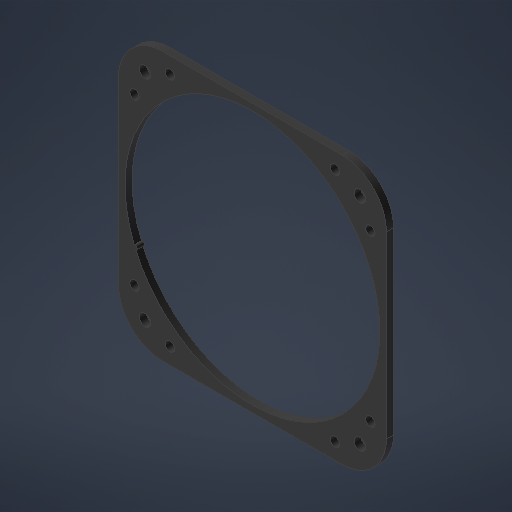
# Autodesk Inventor part: stator_center_00_alu
Saved by Autodesk Inventor 2026.1 (Build 301233000, 233)
## iProperties
Created: 2026-04-12
Part Number: stator_center_00_alu
Material: Generic
Document SubType Name: Modeling
Designer: aaron
Density: 1 g/cm^3
Appearance: Default
Author: aaron
Autodesk Inventor part; units mm, degrees
ref_plane "YZ Plane" through (0, 0, 0) normal (1, 0, 0) x (0, 1, 0)
ref_plane "XZ Plane" through (0, 0, 0) normal (0, 1, 0) x (-1, 0, 0)
ref_plane "XY Plane" through (0, 0, 0) normal (0, 0, 1) x (1, 0, 0)
sketch "Sketch1" plane through (0, 0, 0) normal (0, 0, 1) x (1, 0, 0)
  circle A0 centre (0, 0) radius 57.5
  circle A1 centre (0, 0) radius 60.5
  line L0 (-40.5, 60.5) -> (40.5, 60.5)
  line L1 (60.5, 40.5) -> (60.5, -40.5)
  line L2 (40.5, -60.5) -> (-40.5, -60.5)
  line L3 (-60.5, -40.5) -> (-60.5, 40.5)
  arc A2 (-40.5, 60.5) -> (-60.5, 40.5) centre (-40.5, 40.5) ccw
  arc A3 (60.5, 40.5) -> (40.5, 60.5) centre (40.5, 40.5) ccw
  arc A4 (40.5, -60.5) -> (60.5, -40.5) centre (40.5, -40.5) ccw
  arc A5 (-60.5, -40.5) -> (-40.5, -60.5) centre (-40.5, -40.5) ccw
  dimension "d0" = 115
  dimension "d1" = 121
  dimension "d2" = 20
  constraints: 12 tangent, 8 end point, 8 point on circle, 6 centre point, 3 equal radius, 2 coincident, 2 parallel, 1 horizontal, 1 perpendicular
  measures "d0" diameter of A0
  measures "d1" diameter of A1
  measures "d2" radius of A2
extrude "Extrusion1" add sketch "Sketch1" along normal blind 3.2
sketch "Sketch3" plane through (0, 0, 3.2) normal (0, 0, 1) x (1, 0, 0)
  circle A0 centre (-37.282468, -53.244883) radius 2.15
  circle A1 centre (-48.5, -48.5) radius 2.65
  circle A2 centre (-53.244883, -37.282468) radius 2.15
  circle A3 centre (-53.244883, 37.282468) radius 2.15
  circle A4 centre (-48.5, 48.5) radius 2.65
  circle A5 centre (-37.282468, 53.244883) radius 2.15
  circle A6 centre (37.282468, 53.244883) radius 2.15
  circle A7 centre (48.5, 48.5) radius 2.65
  circle A8 centre (53.244883, 37.282468) radius 2.15
  circle A9 centre (53.244883, -37.282468) radius 2.15
  circle A10 centre (48.5, -48.5) radius 2.65
  circle A11 centre (37.282468, -53.244883) radius 2.15
  point P0 (0, 0)
extrude "Extrusion3" cut sketch "Sketch3" against normal through all
sketch "Sketch4" plane through (0, 0, 3.2) normal (0, 0, 1) x (1, 0, 0)
  arc A0 (-52.049443, -21.979661) -> (-53.351667, -21.444104) centre (-52.970672, -22.368681) ccw
  arc A1 (-52.573656, -23.286493) -> (-52.049443, -21.979661) centre (-52.970672, -22.368681) ccw
  circle A2 centre (-52.970672, -22.368681) radius 0.95
  point P0 (0, 0)
  dimension "d28" = 1.9
  constraints: 1 centre point, 1 coincident
  measures "d28" diameter of A2
extrude "Extrusion4" add sketch "Sketch4" against normal up to surface (3.2 mm away)
sketch "Sketch5" plane through (0, 0, 3.2) normal (0, 0, 1) x (1, 0, 0)
  arc A0 (-52.593886, -23.240766) -> (-53.332999, -21.49049) centre (0, 0) ccw
  circle A1 centre (0, 0) radius 57.55
  arc A2 (-52.593886, -23.240766) -> (-53.332999, -21.49049) centre (-52.970672, -22.368681) ccw
  line L0 (-52.593886, -23.240766) -> (-52.651569, -23.263484)
  line L1 (-53.332999, -21.49049) -> (-53.442689, -21.544242)
  point P0 (-52.640446, -23.259104)
  point P1 (-53.378017, -21.51255)
  dimension "d31" = 0.05
  constraints: 4 end point, 1 centre point, 1 coincident
  measures "d31" radial gap between concentric circles of A0 A1
sketch "Sketch5 outline for Extrusion5" plane through (0, 0, 3.2) normal (0, 0, 1) x (1, 0, 0)
  arc A0 (-53.332999, -21.49049) -> (-52.593886, -23.240766) centre (0, 0) cw
  line L0 (-53.378017, -21.51255) -> (-53.332999, -21.49049)
  arc A1 (-52.640446, -23.259104) -> (-53.378017, -21.51255) centre (0, 0) ccw
  line L1 (-52.593886, -23.240766) -> (-52.640446, -23.259104)
extrude "Extrusion5" cut sketch "Sketch5 outline for Extrusion5" against normal through all
body "Solid1"
